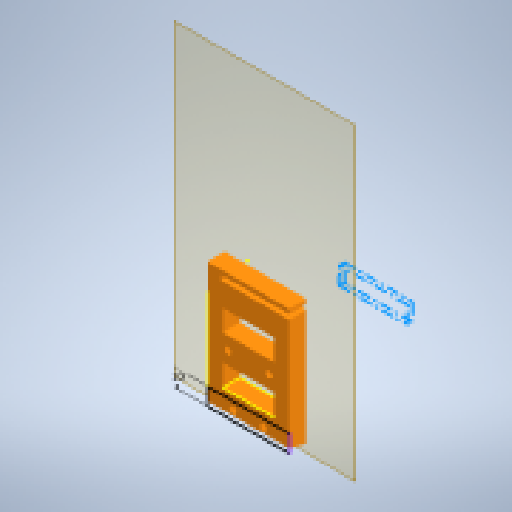
# Autodesk Inventor part: голова
Saved by Autodesk Inventor 2024.2 (Build 282272000, 272)
## iProperties
Created: 2025-10-19
Part Number: голова
Material: PA-CF
Document SubType Name: Modeling
Designer: katya_notebook
Density: 1.18 g/cm^3
Appearance: Оранжевый
Author: katya_notebook
Autodesk Inventor part; units mm, degrees
ref_plane "YZ Plane" through (0, 0, 0) normal (1, 0, 0) x (0, 1, 0)
ref_plane "XZ Plane" through (0, 0, 0) normal (0, 1, 0) x (-1, 0, 0)
ref_plane "XY Plane" through (0, 0, 0) normal (0, 0, 1) x (1, 0, 0)
ref_plane "РабПлоскость1" through (0, 0.0753, 0) normal (0, 0, 1) x (1, 0, 0)
sketch "Эскиз1" plane through (0, 0.0753, 0) normal (0, 0, 1) x (1, 0, 0)
  line L0 (-19.3303, -71.0347) -> (19.3303, -39.116) construction
  line L1 (19.8455, -79.1127) -> (-19.8455, -31.038) construction
  line L2 (24.273, -74.4442) -> (-23.2178, -74.4442)
  line L3 (-23.2178, -74.4442) -> (-23.2178, -26.9534)
  line L4 (-23.2178, -26.9534) -> (24.273, -26.9534)
  line L5 (24.273, -26.9534) -> (24.273, -74.4442)
  line L6 (24.273, -74.4442) -> (-23.2178, -26.9534) construction
  line L7 (-23.2178, -74.4442) -> (24.273, -26.9534) construction
  circle A0 centre (12.4001, -50.6988) radius 2 projected
  circle A1 centre (-11.3449, -50.6988) radius 2 projected
  line L8 (12.4001, -50.6988) -> (-11.3449, -50.6988)
  line L9 (24.273, -26.9534) -> (-23.2178, -26.9534)
  line L10 (-23.2178, -26.9534) -> (-23.2178, -11.4534)
  line L11 (-23.2178, -11.4534) -> (24.273, -11.4534)
  line L12 (24.273, -11.4534) -> (24.273, -26.9534)
  line L13 (-48.4881, -9.5434) -> (12.5836, -9.5434) projected
  point P0 (0, -0.0753)
  point P1 (0, -55.0753)
  point P2 (0.5276, -50.6988)
  dimension "d0" = 40
  dimension "d1" = 40
  dimension "d2" = 55
  dimension "d26" = 47.4908
  dimension "d44" = 15.5
  constraints: 26 end point, 5 midpoint, 4 parallel, 3 horizontal, 3 perpendicular, 1 point on line
  measures "d0" distance of L1.start L0.end
  measures "d1" distance of L0.end L1.end
  measures "d2" distance of point (0, -0.075) point (0, -55.075)
  measures "d26" distance of L4.end L2.start
  measures "d44" distance of L9.end L10.end
extrude "Выдавливание1" add sketch "Эскиз1" along normal blind 10 contours L2 L3 L4 L5 | A0 | A1
sketch "Эскиз5" plane through (0, 0.0753, 10) normal (0, 0, 1) x (1, 0, 0)
  line L0 (-23.2178, -26.9534) -> (-23.2178, -74.4442) projected
  line L1 (-23.2178, -74.4442) -> (24.273, -74.4442)
  line L2 (24.273, -74.4442) -> (24.273, -84.4442)
  line L3 (24.273, -84.4442) -> (-23.2178, -84.4442)
  line L4 (-23.2178, -84.4442) -> (-23.2178, -74.4442)
  point P0 (0, -0.0753)
  dimension "d25" = 10
  constraints: 8 end point, 2 parallel, 1 horizontal, 1 perpendicular
  measures "d25" distance between parallel lines of L3 L1
extrude "Выдавливание5" add sketch "Эскиз5" against normal up to surface (10 mm away)
sketch "Эскиз2" plane through (0, 0.0753, 10) normal (0, 0, 1) x (1, 0, 0)
  line L0 (0.5275, -22.5778) -> (0.5275, -78.8207)
  line L1 (-17.6404, -50.6993) -> (24.2729, -50.6993)
  line L2 (3.3163, -50.6993) -> (-11.345, -50.6993)
  circle A0 centre (-11.345, -50.6993) radius 2
  circle A1 centre (12.4, -50.6993) radius 2
  line L3 (24.273, -26.9534) -> (-23.2178, -26.9534) projected
  line L4 (24.273, -84.4442) -> (24.273, -26.9534) projected
  point P0 (0, -0.0753)
  point P1 (0.5275, -50.6993)
  dimension "d7" = 11.8725
  dimension "d8" = 4
  dimension "d27" = 23.7455
  dimension "d28" = 23.7459
  constraints: 6 end point, 2 centre point, 2 midpoint, 2 parallel, 2 point on line, 1 coincident, 1 horizontal, 1 symmetric about line, 1 other
  measures "d7" distance of point (0.528, -50.699) L2.end
  measures "d8" diameter of A0
  measures "d27" distance between parallel lines of L4 L0
  measures "d28" distance between parallel lines of L3 L1
extrude "Выдавливание2" cut sketch "Эскиз2" against normal blind 10 contours A1 L1 | L1 A1 | L1 A0 | L1 A0
sketch "Эскиз3" plane through (0, 0.0753, 10) normal (0, 0, 1) x (1, 0, 0)
  line L0 (0.5275, -75.4873) -> (0.5275, -27.9965)
  line L1 (-22.6859, -50.6993) -> (23.741, -50.6993)
  line L2 (15.5275, -70.6951) -> (-14.4725, -70.6951)
  line L3 (-14.4725, -70.6951) -> (-14.4725, -58.1951)
  line L4 (-14.4725, -58.1951) -> (15.5275, -58.1951)
  line L5 (15.5275, -58.1951) -> (15.5275, -70.6951)
  line L6 (15.5275, -70.6951) -> (-14.4725, -58.1951) construction
  line L7 (-14.4725, -70.6951) -> (15.5275, -58.1951) construction
  line L8 (-14.4725, -43.2034) -> (15.5275, -43.2034)
  line L9 (15.5275, -43.2034) -> (15.5275, -30.7034)
  line L10 (15.5275, -30.7034) -> (-14.4725, -30.7034)
  line L11 (-14.4725, -30.7034) -> (-14.4725, -43.2034)
  line L12 (-14.4725, -43.2034) -> (15.5275, -30.7034) construction
  line L13 (15.5275, -43.2034) -> (-14.4725, -30.7034) construction
  line L14 (24.273, -26.9534) -> (-23.2178, -26.9534) projected
  line L15 (24.273, -84.4442) -> (24.273, -26.9534) projected
  line L16 (24.273, -74.4451) -> (-23.2178, -74.4451)
  line L17 (-23.2178, -26.9534) -> (-23.2178, -84.4442) projected
  point P0 (0, -0.0753)
  point P1 (0.5275, -64.4451)
  point P2 (0.5275, -74.4451)
  point P3 (0.5275, -50.6993)
  point P4 (0.5275, -36.9534)
  dimension "d11" = 30
  dimension "d12" = 12.5
  dimension "d13" = 10
  dimension "d29" = 23.7455
  dimension "d30" = 23.7459
  dimension "d31" = 10
  dimension "d32" = 23.7459
  dimension "d33" = 10
  constraints: 30 end point, 6 parallel, 5 midpoint, 5 point on line, 3 horizontal, 2 equal length, 2 perpendicular
  measures "d11" distance of L3.end L4.end
  measures "d12" distance of L4.end L2.start
  measures "d13" distance of point (0.528, -74.445) point (0.528, -64.445)
  measures "d29" distance from line of L15 point (0.528, -50.699)
  measures "d30" distance between parallel lines of L14 L1
  measures "d31" distance from line of L14 point (0.528, -36.953)
  measures "d32" distance between parallel lines of L1 L16
  measures "d33" distance from line of L16 point (0.528, -64.445)
extrude "Выдавливание3" cut sketch "Эскиз3" against normal blind 10 contours L2 L3 L4 L0 | L0 L4 L5 L2 | L8 L11 L10 L0 | L0 L10 L9 L8
sketch "Эскиз4" plane through (-14.4725, -70.6198, 10) normal (0, 1, 0) x (1, 0, 0)
  line L0 (30, 0) -> (0, 0) projected
  line L1 (30, 0) -> (30, 10) projected
  line L2 (0, 10) -> (30, 10) projected
  line L3 (0, 0) -> (0, 10) projected
ref_plane "РабПлоскость2" through (-14.9975, -72.9954, 9.931) normal (0.0042784, 0.9999908, 0) x (0, 0, 1)
sketch "Эскиз6" plane through (0, 0.0753, 10) normal (0, 0, 1) x (1, 0, 0)
  line L0 (-14.9724, -74.9534) -> (-29.9724, -74.9534) projected
  circle A0 centre (-8.2178, -78.9534) radius 2
  circle A1 centre (9.273, -78.9534) radius 2
  line L1 (-23.2178, -26.9534) -> (-23.2178, -84.4442) projected
  line L2 (24.273, -84.4442) -> (24.273, -26.9534) projected
  point P0 (0, -0.0753)
  dimension "d34" = 4
  dimension "d35" = 4
  dimension "d36" = 15
  dimension "d37" = 15
  dimension "d38" = 4
  constraints: 2 centre point, 1 equal radius
  measures "d34" diameter of A1
  measures "d35" distance from line of L0 A0.centre
  measures "d36" distance from line of A0.centre L1
  measures "d37" distance from line of L2 A1.centre
  measures "d38" distance from line of L0 A1.centre
extrude "Выдавливание6" cut sketch "Эскиз6" against normal blind 10
sketch "Эскиз7" plane through (-23.2178, -26.8781, 0) normal (-1, 0, 0) x (0, 0, 1)
  line L0 (10, -50) -> (10, -54) projected
  line L1 (10, -55) -> (0, -57.4908)
  line L2 (10, -55) -> (14.1948, -61.9717)
  line L3 (0.2707, -57.4234) -> (14.1948, -61.9717)
  point P0 (0, 26.8781)
  point P1 (0, -57.4908)
  dimension "d41" = 1
  constraints: 6 end point, 1 coincident, 1 point on line
  measures "d41" distance of L1.start L0.end
extrude "Выдавливание7" cut sketch "Эскиз7" against normal blind 74.25
sketch "Эскиз8" plane through (-23.2178, -26.8781, 0) normal (0, 1, 0) x (1, 0, 0)
  line L0 (47.4908, 0) -> (47.4908, -10) projected
  line L1 (47.4908, 0) -> (0, 0) projected
  line L2 (47.4908, -10) -> (0, -10) projected
  line L3 (0, 0) -> (0, -10) projected
  point P0 (23.2178, 0)
extrude "Выдавливание8" add sketch "Эскиз8" along normal blind 15
sketch "Эскиз9" plane through (0, 0.0753, 10) normal (0, 0, 1) x (1, 0, 0)
  line L0 (25.5767, -17.4448) -> (-15.3378, -17.4448) projected
  line L1 (25.5767, -14.5434) -> (25.5767, -17.4448) projected
  line L2 (20.4005, -12.5434) -> (12.5836, -12.5434) projected
  line L3 (-15.3378, -17.4448) -> (-15.3378, -14.5434) projected
  line L4 (-15.3378, -14.5434) -> (25.5767, -14.5434) projected
  line L5 (21.6487, -17.4448) -> (21.6487, -14.5434)
  point P0 (0, -0.0753)
  constraints: 2 end point, 2 point on line, 1 vertical
extrude "Выдавливание9" cut sketch "Эскиз9" against normal blind 15 contours L0 L3 L4 L5
